Autodesk Fusion 360 part; units mm, degrees
(part 7 of 8)
  spline S189 degree 5 poles (12.6796, 61.4083) (12.6796, 61.409) (12.6791, 61.4272) (12.6782, 61.4629) (12.6766, 61.5161) (12.6742, 61.5869) (12.6707, 61.6745) (12.6667, 61.7622) (12.6623, 61.8499) (12.6573, 61.9376) (12.6519, 62.0254) (12.646, 62.1133) (12.6396, 62.2012) (12.6327, 62.2891) (12.6255, 62.3771) (12.6177, 62.4651) (12.6096, 62.5532) (12.601, 62.6413) (12.592, 62.7294) (12.5826, 62.8175) (12.5727, 62.9057) (12.5625, 62.9939) (12.5519, 63.0822) (12.5408, 63.1704) (12.5294, 63.2587) (12.5175, 63.347) (12.5053, 63.4353) (12.4927, 63.5237) (12.4798, 63.612) (12.4664, 63.7004) (12.4527, 63.7888) (12.4386, 63.8772) (12.4242, 63.9657) (12.4093, 64.0541) (12.3942, 64.1426) (12.3787, 64.231) (12.3628, 64.3195) (12.3466, 64.408) (12.33, 64.4965) (12.3131, 64.585) (12.2958, 64.6735) (12.2782, 64.762) (12.2603, 64.8506) (12.242, 64.9391) (12.2234, 65.0276) (12.2045, 65.1162) (12.1852, 65.2047) (12.1656, 65.2933) (12.1457, 65.3818) (12.1255, 65.4703) (12.1049, 65.5589) (12.0841, 65.6474) (12.0629, 65.736) (12.0457, 65.8068) (12.0327, 65.8599) (12.0239, 65.8954) (12.0195, 65.9131) knots 0.270845 0.270845 0.270845 0.270845 0.270845 0.270845 0.271429 0.285714 0.3 0.314286 0.328571 0.342857 0.357143 0.371429 0.385714 0.4 0.414286 0.428571 0.442857 0.457143 0.471429 0.485714 0.5 0.514286 0.528571 0.542857 0.557143 0.571429 0.585714 0.6 0.614286 0.628571 0.642857 0.657143 0.671429 0.685714 0.7 0.714286 0.728571 0.742857 0.757143 0.771429 0.785714 0.8 0.814286 0.828571 0.842857 0.857143 0.871429 0.885714 0.9 0.914286 0.928571 0.942857 0.957143 0.971429 0.985714 1 1 1 1 1 1
  arc A95 (12.0195, 65.9131) -> (10.5389, 66.1659) centre (0, 0) ccw
  spline S190 degree 5 poles (10.5389, 66.1659) (10.5289, 66.1507) (10.5089, 66.1202) (10.4789, 66.0744) (10.4392, 66.0133) (10.3898, 65.9368) (10.3408, 65.8602) (10.292, 65.7835) (10.2435, 65.7067) (10.1954, 65.6298) (10.1475, 65.5527) (10.0999, 65.4756) (10.0527, 65.3984) (10.0058, 65.321) (9.9592, 65.2436) (9.9129, 65.166) (9.8669, 65.0884) (9.8212, 65.0106) (9.7759, 64.9327) (9.7309, 64.8547) (9.6862, 64.7766) (9.6418, 64.6985) (9.5978, 64.6202) (9.5542, 64.5417) (9.5108, 64.4632) (9.4679, 64.3846) (9.4252, 64.3059) (9.3829, 64.227) (9.341, 64.1481) (9.2995, 64.0691) (9.2583, 63.9899) (9.2174, 63.9106) (9.177, 63.8313) (9.1369, 63.7518) (9.0971, 63.6722) (9.0578, 63.5925) (9.0189, 63.5127) (8.9803, 63.4328) (8.9422, 63.3528) (8.9045, 63.2726) (8.8671, 63.1924) (8.8302, 63.112) (8.7937, 63.0316) (8.7576, 62.951) (8.722, 62.8703) (8.6868, 62.7895) (8.6521, 62.7086) (8.6178, 62.6276) (8.584, 62.5464) (8.5507, 62.4652) (8.5178, 62.3838) (8.4854, 62.3023) (8.4597, 62.2363) (8.4406, 62.1867) (8.4278, 62.1533) (8.4213, 62.1363) (8.4211, 62.1356) knots -1 -1 -1 -1 -1 -1 -0.985714 -0.971429 -0.957143 -0.942857 -0.928571 -0.914286 -0.9 -0.885714 -0.871429 -0.857143 -0.842857 -0.828571 -0.814286 -0.8 -0.785714 -0.771429 -0.757143 -0.742857 -0.728571 -0.714286 -0.7 -0.685714 -0.671429 -0.657143 -0.642857 -0.628571 -0.614286 -0.6 -0.585714 -0.571429 -0.557143 -0.542857 -0.528571 -0.514286 -0.5 -0.485714 -0.471429 -0.457143 -0.442857 -0.428571 -0.414286 -0.4 -0.385714 -0.371429 -0.357143 -0.342857 -0.328571 -0.314286 -0.3 -0.285714 -0.271429 -0.270845 -0.270845 -0.270845 -0.270845 -0.270845 -0.270845
  spline S191 degree 3 poles (8.2079, 62.0083) (8.2337, 62.0049) (8.2599, 62.0066) (8.3103, 62.0199) (8.3339, 62.0313) (8.3696, 62.0583) (8.3829, 62.0717) (8.4054, 62.1016) (8.4144, 62.1181) (8.4211, 62.1356) knots 0 0 0 0 0.007813 0.007813 0.015626 0.015626 0.021241 0.021241 0.026855 0.026855 0.026855 0.026855
  arc A96 (8.2079, 62.0083) -> (6.8702, 62.1708) centre (0, 0) ccw
  spline S192 degree 3 poles (6.6936, 62.3453) (6.6968, 62.3195) (6.705, 62.2945) (6.7304, 62.2491) (6.7475, 62.229) (6.7825, 62.2012) (6.7988, 62.1917) (6.8334, 62.1775) (6.8516, 62.1728) (6.8702, 62.1708) knots 0 0 0 0 0.007813 0.007813 0.015626 0.015626 0.021241 0.021241 0.026855 0.026855 0.026855 0.026855
  spline S193 degree 5 poles (6.6936, 62.3453) (6.6935, 62.346) (6.6913, 62.3641) (6.687, 62.3996) (6.6803, 62.4524) (6.671, 62.5226) (6.6591, 62.6095) (6.6467, 62.6963) (6.6338, 62.7832) (6.6204, 62.8701) (6.6065, 62.957) (6.5921, 63.0438) (6.5773, 63.1307) (6.562, 63.2176) (6.5463, 63.3045) (6.5301, 63.3913) (6.5135, 63.4782) (6.4964, 63.565) (6.479, 63.6519) (6.4611, 63.7387) (6.4428, 63.8255) (6.4241, 63.9123) (6.405, 63.9991) (6.3854, 64.0859) (6.3655, 64.1726) (6.3452, 64.2594) (6.3246, 64.3461) (6.3035, 64.4328) (6.2821, 64.5195) (6.2602, 64.6062) (6.2381, 64.6929) (6.2155, 64.7795) (6.1926, 64.8661) (6.1693, 64.9527) (6.1457, 65.0393) (6.1217, 65.1259) (6.0973, 65.2124) (6.0726, 65.2989) (6.0476, 65.3854) (6.0222, 65.4719) (5.9965, 65.5583) (5.9704, 65.6447) (5.9441, 65.7311) (5.9173, 65.8175) (5.8903, 65.9038) (5.8629, 65.9901) (5.8352, 66.0764) (5.8071, 66.1626) (5.7788, 66.2488) (5.7501, 66.335) (5.7211, 66.4211) (5.6918, 66.5073) (5.6621, 66.5933) (5.6382, 66.6622) (5.6201, 66.7138) (5.608, 66.7482) (5.6019, 66.7654) knots 0.270845 0.270845 0.270845 0.270845 0.270845 0.270845 0.271429 0.285714 0.3 0.314286 0.328571 0.342857 0.357143 0.371429 0.385714 0.4 0.414286 0.428571 0.442857 0.457143 0.471429 0.485714 0.5 0.514286 0.528571 0.542857 0.557143 0.571429 0.585714 0.6 0.614286 0.628571 0.642857 0.657143 0.671429 0.685714 0.7 0.714286 0.728571 0.742857 0.757143 0.771429 0.785714 0.8 0.814286 0.828571 0.842857 0.857143 0.871429 0.885714 0.9 0.914286 0.928571 0.942857 0.957143 0.971429 0.985714 1 1 1 1 1 1
  arc A97 (5.6019, 66.7654) -> (4.1038, 66.8742) centre (0, 0) ccw
  spline S194 degree 5 poles (4.1038, 66.8742) (4.0953, 66.8581) (4.0783, 66.8258) (4.0529, 66.7773) (4.0193, 66.7127) (3.9775, 66.6318) (3.9361, 66.5508) (3.8949, 66.4697) (3.8541, 66.3886) (3.8136, 66.3074) (3.7734, 66.2261) (3.7335, 66.1447) (3.6939, 66.0633) (3.6547, 65.9818) (3.6157, 65.9002) (3.5771, 65.8185) (3.5389, 65.7368) (3.5009, 65.655) (3.4633, 65.5731) (3.4261, 65.4911) (3.3891, 65.4091) (3.3525, 65.327) (3.3163, 65.2448) (3.2804, 65.1626) (3.2448, 65.0802) (3.2097, 64.9978) (3.1748, 64.9153) (3.1403, 64.8328) (3.1062, 64.7502) (3.0725, 64.6675) (3.0391, 64.5847) (3.0061, 64.5019) (2.9735, 64.419) (2.9413, 64.336) (2.9094, 64.253) (2.878, 64.1698) (2.8469, 64.0866) (2.8163, 64.0034) (2.786, 63.9201) (2.7562, 63.8367) (2.7268, 63.7532) (2.6978, 63.6696) (2.6692, 63.586) (2.6411, 63.5024) (2.6134, 63.4186) (2.5862, 63.3348) (2.5594, 63.2509) (2.5331, 63.1669) (2.5073, 63.0829) (2.482, 62.9988) (2.4571, 62.9146) (2.4328, 62.8304) (2.4135, 62.7623) (2.3993, 62.711) (2.3898, 62.6765) (2.385, 62.659) (2.3848, 62.6583) knots -1 -1 -1 -1 -1 -1 -0.985714 -0.971429 -0.957143 -0.942857 -0.928571 -0.914286 -0.9 -0.885714 -0.871429 -0.857143 -0.842857 -0.828571 -0.814286 -0.8 -0.785714 -0.771429 -0.757143 -0.742857 -0.728571 -0.714286 -0.7 -0.685714 -0.671429 -0.657143 -0.642857 -0.628571 -0.614286 -0.6 -0.585714 -0.571429 -0.557143 -0.542857 -0.528571 -0.514286 -0.5 -0.485714 -0.471429 -0.457143 -0.442857 -0.428571 -0.414286 -0.4 -0.385714 -0.371429 -0.357143 -0.342857 -0.328571 -0.314286 -0.3 -0.285714 -0.271429 -0.270845 -0.270845 -0.270845 -0.270845 -0.270845 -0.270845
  spline S195 degree 3 poles (2.1849, 62.511) (2.2109, 62.5101) (2.2369, 62.5143) (2.2857, 62.5324) (2.3081, 62.5461) (2.3411, 62.5764) (2.353, 62.591) (2.3725, 62.6229) (2.3799, 62.6402) (2.3848, 62.6583) knots 0 0 0 0 0.007813 0.007813 0.015626 0.015626 0.021241 0.021241 0.026855 0.026855 0.026855 0.026855
  arc A98 (2.1849, 62.511) -> (0.8378, 62.5436) centre (0, 0) ccw
  spline S196 degree 3 poles (0.6452, 62.7003) (0.6508, 62.6749) (0.6614, 62.6508) (0.6911, 62.608) (0.71, 62.5898) (0.7476, 62.5655) (0.7646, 62.5576) (0.8005, 62.5467) (0.8191, 62.5438) (0.8378, 62.5436) knots 0 0 0 0 0.007813 0.007813 0.015626 0.015626 0.021241 0.021241 0.026855 0.026855 0.026855 0.026855
  spline S197 degree 5 poles (0.6452, 62.7003) (0.645, 62.701) (0.6411, 62.7188) (0.6333, 62.7537) (0.6215, 62.8056) (0.6056, 62.8746) (0.5853, 62.9599) (0.5646, 63.0452) (0.5434, 63.1304) (0.5216, 63.2156) (0.4994, 63.3007) (0.4767, 63.3858) (0.4536, 63.4708) (0.43, 63.5558) (0.4059, 63.6407) (0.3815, 63.7256) (0.3565, 63.8105) (0.3312, 63.8953) (0.3054, 63.98) (0.2792, 64.0647) (0.2526, 64.1494) (0.2257, 64.2339) (0.1983, 64.3185) (0.1705, 64.403) (0.1423, 64.4874) (0.1137, 64.5718) (0.0847, 64.6561) (0.0554, 64.7404) (0.0257, 64.8246) (-0.0044, 64.9088) (-0.0348, 64.9929) (-0.0656, 65.077) (-0.0968, 65.161) (-0.1283, 65.2449) (-0.1602, 65.3288) (-0.1925, 65.4127) (-0.225, 65.4965) (-0.258, 65.5802) (-0.2912, 65.6638) (-0.3248, 65.7475) (-0.3588, 65.831) (-0.3931, 65.9145) (-0.4277, 65.9979) (-0.4626, 66.0813) (-0.4979, 66.1646) (-0.5335, 66.2479) (-0.5694, 66.3311) (-0.6056, 66.4142) (-0.6421, 66.4973) (-0.679, 66.5803) (-0.7162, 66.6632) (-0.7537, 66.7461) (-0.7915, 66.8289) (-0.822, 66.8951) (-0.845, 66.9448) (-0.8604, 66.9778) (-0.8681, 66.9944) knots 0.270845 0.270845 0.270845 0.270845 0.270845 0.270845 0.271429 0.285714 0.3 0.314286 0.328571 0.342857 0.357143 0.371429 0.385714 0.4 0.414286 0.428571 0.442857 0.457143 0.471429 0.485714 0.5 0.514286 0.528571 0.542857 0.557143 0.571429 0.585714 0.6 0.614286 0.628571 0.642857 0.657143 0.671429 0.685714 0.7 0.714286 0.728571 0.742857 0.757143 0.771429 0.785714 0.8 0.814286 0.828571 0.842857 0.857143 0.871429 0.885714 0.9 0.914286 0.928571 0.942857 0.957143 0.971429 0.985714 1 1 1 1 1 1
  arc A99 (-0.8681, 66.9944) -> (-2.3697, 66.9581) centre (0, 0) ccw
  spline S198 degree 5 poles (-2.3697, 66.9581) (-2.3766, 66.9412) (-2.3904, 66.9074) (-2.4109, 66.8567) (-2.4382, 66.7891) (-2.4719, 66.7046) (-2.5054, 66.62) (-2.5385, 66.5353) (-2.5713, 66.4506) (-2.6038, 66.3659) (-2.636, 66.2811) (-2.6678, 66.1963) (-2.6994, 66.1114) (-2.7306, 66.0265) (-2.7614, 65.9415) (-2.792, 65.8565) (-2.8222, 65.7715) (-2.852, 65.6864) (-2.8816, 65.6012) (-2.9107, 65.5161) (-2.9396, 65.4308) (-2.9681, 65.3456) (-2.9962, 65.2603) (-3.024, 65.175) (-3.0515, 65.0896) (-3.0785, 65.0042) (-3.1052, 64.9187) (-3.1316, 64.8332) (-3.1576, 64.7477) (-3.1832, 64.6621) (-3.2084, 64.5765) (-3.2332, 64.4909) (-3.2577, 64.4052) (-3.2818, 64.3195) (-3.3055, 64.2338) (-3.3287, 64.148) (-3.3516, 64.0622) (-3.3741, 63.9764) (-3.3962, 63.8905) (-3.4178, 63.8047) (-3.439, 63.7187) (-3.4598, 63.6328) (-3.4802, 63.5468) (-3.5001, 63.4608) (-3.5196, 63.3748) (-3.5386, 63.2887) (-3.5571, 63.2026) (-3.5752, 63.1165) (-3.5928, 63.0304) (-3.6099, 62.9443) (-3.6265, 62.8581) (-3.6426, 62.7719) (-3.6552, 62.7022) (-3.6644, 62.6498) (-3.6705, 62.6146) (-3.6736, 62.5966) (-3.6737, 62.5959) knots -1 -1 -1 -1 -1 -1 -0.985714 -0.971429 -0.957143 -0.942857 -0.928571 -0.914286 -0.9 -0.885714 -0.871429 -0.857143 -0.842857 -0.828571 -0.814286 -0.8 -0.785714 -0.771429 -0.757143 -0.742857 -0.728571 -0.714286 -0.7 -0.685714 -0.671429 -0.657143 -0.642857 -0.628571 -0.614286 -0.6 -0.585714 -0.571429 -0.557143 -0.542857 -0.528571 -0.514286 -0.5 -0.485714 -0.471429 -0.457143 -0.442857 -0.428571 -0.414286 -0.4 -0.385714 -0.371429 -0.357143 -0.342857 -0.328571 -0.314286 -0.3 -0.285714 -0.271429 -0.270845 -0.270845 -0.270845 -0.270845 -0.270845 -0.270845
  spline S199 degree 3 poles (-3.8585, 62.4301) (-3.8325, 62.4317) (-3.8071, 62.4384) (-3.7602, 62.4611) (-3.7392, 62.4769) (-3.7093, 62.5102) (-3.6989, 62.5259) (-3.6826, 62.5596) (-3.6769, 62.5775) (-3.6737, 62.5959) knots 0 0 0 0 0.007813 0.007813 0.015626 0.015626 0.021241 0.021241 0.026855 0.026855 0.026855 0.026855
  arc A100 (-3.8585, 62.4301) -> (-5.2025, 62.3325) centre (0, 0) ccw
  spline S200 degree 3 poles (-5.4093, 62.4699) (-5.4012, 62.4451) (-5.3884, 62.4222) (-5.3547, 62.3825) (-5.3341, 62.3661) (-5.2943, 62.3455) (-5.2766, 62.3393) (-5.2399, 62.332) (-5.2211, 62.3309) (-5.2025, 62.3325) knots 0 0 0 0 0.007813 0.007813 0.015626 0.015626 0.021241 0.021241 0.026855 0.026855 0.026855 0.026855
  spline S201 degree 5 poles (-5.4093, 62.4699) (-5.4095, 62.4706) (-5.4151, 62.4879) (-5.4262, 62.5218) (-5.443, 62.5724) (-5.4655, 62.6395) (-5.4939, 62.7225) (-5.5228, 62.8053) (-5.5521, 62.8881) (-5.582, 62.9708) (-5.6123, 63.0534) (-5.6431, 63.1359) (-5.6743, 63.2183) (-5.706, 63.3006) (-5.7382, 63.3828) (-5.7707, 63.465) (-5.8037, 63.547) (-5.8371, 63.6289) (-5.871, 63.7108) (-5.9052, 63.7926) (-5.9398, 63.8743) (-5.9749, 63.9559) (-6.0103, 64.0374) (-6.0461, 64.1188) (-6.0823, 64.2001) (-6.1189, 64.2813) (-6.1559, 64.3625) (-6.1932, 64.4435) (-6.2309, 64.5245) (-6.269, 64.6054) (-6.3074, 64.6862) (-6.3462, 64.7668) (-6.3853, 64.8475) (-6.4248, 64.928) (-6.4646, 65.0084) (-6.5048, 65.0887) (-6.5453, 65.169) (-6.5862, 65.2491) (-6.6273, 65.3292) (-6.6689, 65.4092) (-6.7107, 65.4891) (-6.7529, 65.5688) (-6.7954, 65.6485) (-6.8382, 65.7282) (-6.8813, 65.8077) (-6.9248, 65.8871) (-6.9686, 65.9665) (-7.0127, 66.0457) (-7.0571, 66.1249) (-7.1018, 66.2039) (-7.1468, 66.2829) (-7.1921, 66.3618) (-7.2377, 66.4406) (-7.2744, 66.5035) (-7.3021, 66.5507) (-7.3206, 66.5821) (-7.3299, 66.5978) knots 0.270845 0.270845 0.270845 0.270845 0.270845 0.270845 0.271429 0.285714 0.3 0.314286 0.328571 0.342857 0.357143 0.371429 0.385714 0.4 0.414286 0.428571 0.442857 0.457143 0.471429 0.485714 0.5 0.514286 0.528571 0.542857 0.557143 0.571429 0.585714 0.6 0.614286 0.628571 0.642857 0.657143 0.671429 0.685714 0.7 0.714286 0.728571 0.742857 0.757143 0.771429 0.785714 0.8 0.814286 0.828571 0.842857 0.857143 0.871429 0.885714 0.9 0.914286 0.928571 0.942857 0.957143 0.971429 0.985714 1 1 1 1 1 1
  arc A101 (-7.3299, 66.5978) -> (-8.821, 66.4168) centre (0, 0) ccw
  spline S202 degree 5 poles (-8.821, 66.4168) (-8.8262, 66.3993) (-8.8367, 66.3644) (-8.8523, 66.3119) (-8.8729, 66.242) (-8.8983, 66.1546) (-8.9234, 66.0672) (-8.9482, 65.9797) (-8.9727, 65.8923) (-8.9969, 65.8048) (-9.0207, 65.7173) (-9.0442, 65.6298) (-9.0674, 65.5422) (-9.0903, 65.4547) (-9.1128, 65.3672) (-9.135, 65.2796) (-9.1568, 65.192) (-9.1784, 65.1045) (-9.1995, 65.0169) (-9.2204, 64.9293) (-9.2408, 64.8417) (-9.261, 64.7541) (-9.2808, 64.6665) (-9.3002, 64.5788) (-9.3193, 64.4912) (-9.338, 64.4036) (-9.3563, 64.3159) (-9.3743, 64.2283) (-9.3919, 64.1407) (-9.4091, 64.053) (-9.426, 63.9654) (-9.4424, 63.8778) (-9.4585, 63.7902) (-9.4742, 63.7025) (-9.4895, 63.6149) (-9.5044, 63.5273) (-9.5189, 63.4397) (-9.533, 63.3521) (-9.5466, 63.2645) (-9.5599, 63.1769) (-9.5727, 63.0894) (-9.5851, 63.0018) (-9.5971, 62.9143) (-9.6086, 62.8267) (-9.6197, 62.7392) (-9.6303, 62.6517) (-9.6404, 62.5643) (-9.6501, 62.4768) (-9.6593, 62.3894) (-9.668, 62.302) (-9.6762, 62.2146) (-9.6839, 62.1273) (-9.6897, 62.0567) (-9.6939, 62.0036) (-9.6965, 61.968) (-9.6979, 61.9499) (-9.6979, 61.9491) knots -1 -1 -1 -1 -1 -1 -0.985714 -0.971429 -0.957143 -0.942857 -0.928571 -0.914286 -0.9 -0.885714 -0.871429 -0.857143 -0.842857 -0.828571 -0.814286 -0.8 -0.785714 -0.771429 -0.757143 -0.742857 -0.728571 -0.714286 -0.7 -0.685714 -0.671429 -0.657143 -0.642857 -0.628571 -0.614286 -0.6 -0.585714 -0.571429 -0.557143 -0.542857 -0.528571 -0.514286 -0.5 -0.485714 -0.471429 -0.457143 -0.442857 -0.428571 -0.414286 -0.4 -0.385714 -0.371429 -0.357143 -0.342857 -0.328571 -0.314286 -0.3 -0.285714 -0.271429 -0.270845 -0.270845 -0.270845 -0.270845 -0.270845 -0.270845
  spline S203 degree 3 poles (-9.8659, 61.7662) (-9.8401, 61.7703) (-9.8155, 61.7794) (-9.771, 61.8066) (-9.7516, 61.8243) (-9.7251, 61.8604) (-9.7162, 61.877) (-9.7033, 61.9121) (-9.6993, 61.9305) (-9.6979, 61.9491) knots 0 0 0 0 0.007813 0.007813 0.015626 0.015626 0.021241 0.021241 0.026855 0.026855 0.026855 0.026855
  arc A102 (-9.8659, 61.7662) -> (-11.1941, 61.5394) centre (0, 0) ccw
  spline S204 degree 3 poles (-11.4132, 61.6562) (-11.4028, 61.6323) (-11.3878, 61.6107) (-11.3505, 61.5744) (-11.3284, 61.5601) (-11.2868, 61.5435) (-11.2686, 61.539) (-11.2313, 61.5353) (-11.2125, 61.536) (-11.1941, 61.5394) knots 0 0 0 0 0.007813 0.007813 0.015626 0.015626 0.021241 0.021241 0.026855 0.026855 0.026855 0.026855
  spline S205 degree 5 poles (-11.4132, 61.6562) (-11.4135, 61.6568) (-11.4208, 61.6735) (-11.4351, 61.7062) (-11.4567, 61.7549) (-11.4856, 61.8196) (-11.5218, 61.8994) (-11.5586, 61.9791) (-11.5958, 62.0587) (-11.6335, 62.1381) (-11.6716, 62.2174) (-11.7102, 62.2965) (-11.7493, 62.3755) (-11.7888, 62.4544) (-11.8287, 62.5331) (-11.869, 62.6117) (-11.9098, 62.6902) (-11.951, 62.7685) (-11.9925, 62.8468) (-12.0345, 62.9248) (-12.0769, 63.0028) (-12.1196, 63.0806) (-12.1627, 63.1583) (-12.2063, 63.2359) (-12.2501, 63.3134) (-12.2944, 63.3907) (-12.339, 63.4679) (-12.384, 63.545) (-12.4293, 63.6219) (-12.475, 63.6987) (-12.5211, 63.7754) (-12.5674, 63.852) (-12.6142, 63.9285) (-12.6612, 64.0048) (-12.7087, 64.081) (-12.7564, 64.1571) (-12.8045, 64.233) (-12.8529, 64.3089) (-12.9016, 64.3846) (-12.9506, 64.4602) (-13, 64.5356) (-13.0497, 64.611) (-13.0997, 64.6862) (-13.15, 64.7613) (-13.2006, 64.8363) (-13.2515, 64.9112) (-13.3027, 64.9859) (-13.3543, 65.0606) (-13.4061, 65.1351) (-13.4582, 65.2094) (-13.5106, 65.2837) (-13.5633, 65.3578) (-13.6163, 65.4319) (-13.659, 65.491) (-13.6911, 65.5353) (-13.7126, 65.5648) (-13.7233, 65.5795) knots 0.270845 0.270845 0.270845 0.270845 0.270845 0.270845 0.271429 0.285714 0.3 0.314286 0.328571 0.342857 0.357143 0.371429 0.385714 0.4 0.414286 0.428571 0.442857 0.457143 0.471429 0.485714 0.5 0.514286 0.528571 0.542857 0.557143 0.571429 0.585714 0.6 0.614286 0.628571 0.642857 0.657143 0.671429 0.685714 0.7 0.714286 0.728571 0.742857 0.757143 0.771429 0.785714 0.8 0.814286 0.828571 0.842857 0.857143 0.871429 0.885714 0.9 0.914286 0.928571 0.942857 0.957143 0.971429 0.985714 1 1 1 1 1 1
  arc A103 (-13.7233, 65.5795) -> (-15.19, 65.2554) centre (0, 0) ccw
  spline S206 degree 5 poles (-15.19, 65.2554) (-15.1935, 65.2375) (-15.2005, 65.2017) (-15.211, 65.148) (-15.2247, 65.0764) (-15.2416, 64.987) (-15.2582, 64.8975) (-15.2744, 64.8081) (-15.2903, 64.7187) (-15.306, 64.6292) (-15.3212, 64.5399) (-15.3362, 64.4505) (-15.3508, 64.3611) (-15.3651, 64.2718) (-15.3791, 64.1825) (-15.3927, 64.0932) (-15.406, 64.0039) (-15.419, 63.9147) (-15.4316, 63.8255) (-15.4439, 63.7363) (-15.4558, 63.6471) (-15.4674, 63.558) (-15.4786, 63.4688) (-15.4895, 63.3798) (-15.5, 63.2907) (-15.5102, 63.2017) (-15.52, 63.1127) (-15.5294, 63.0237) (-15.5385, 62.9348) (-15.5472, 62.8459) (-15.5555, 62.7571) (-15.5634, 62.6683) (-15.571, 62.5795) (-15.5781, 62.4908) (-15.5849, 62.4021) (-15.5913, 62.3134) (-15.5973, 62.2248) (-15.6028, 62.1363) (-15.608, 62.0478) (-15.6127, 61.9593) (-15.617, 61.8709) (-15.6209, 61.7826) (-15.6244, 61.6943) (-15.6274, 61.6061) (-15.63, 61.5179) (-15.6321, 61.4298) (-15.6338, 61.3418) (-15.6349, 61.2538) (-15.6357, 61.1659) (-15.6359, 61.0781) (-15.6356, 60.9903) (-15.6349, 60.9026) (-15.6338, 60.8318) (-15.6328, 60.7786) (-15.6321, 60.7429) (-15.6316, 60.7247) (-15.6316, 60.724) knots -1 -1 -1 -1 -1 -1 -0.985714 -0.971429 -0.957143 -0.942857 -0.928571 -0.914286 -0.9 -0.885714 -0.871429 -0.857143 -0.842857 -0.828571 -0.814286 -0.8 -0.785714 -0.771429 -0.757143 -0.742857 -0.728571 -0.714286 -0.7 -0.685714 -0.671429 -0.657143 -0.642857 -0.628571 -0.614286 -0.6 -0.585714 -0.571429 -0.557143 -0.542857 -0.528571 -0.514286 -0.5 -0.485714 -0.471429 -0.457143 -0.442857 -0.428571 -0.414286 -0.4 -0.385714 -0.371429 -0.357143 -0.342857 -0.328571 -0.314286 -0.3 -0.285714 -0.271429 -0.270845 -0.270845 -0.270845 -0.270845 -0.270845 -0.270845
  spline S207 degree 3 poles (-15.7811, 60.5257) (-15.7559, 60.5323) (-15.7322, 60.5437) (-15.6906, 60.575) (-15.673, 60.5945) (-15.6501, 60.633) (-15.6429, 60.6504) (-15.6334, 60.6866) (-15.6312, 60.7052) (-15.6316, 60.724) knots 0 0 0 0 0.007813 0.007813 0.015626 0.015626 0.021241 0.021241 0.026855 0.026855 0.026855 0.026855
  arc A104 (-15.7811, 60.5257) -> (-17.0813, 60.1717) centre (0, 0) ccw
  spline S208 degree 3 poles (-17.3106, 60.2668) (-17.298, 60.244) (-17.281, 60.224) (-17.2403, 60.1915) (-17.2169, 60.1794) (-17.174, 60.1669) (-17.1553, 60.1642) (-17.1179, 60.164) (-17.0993, 60.1666) (-17.0813, 60.1717) knots 0 0 0 0 0.007813 0.007813 0.015626 0.015626 0.021241 0.021241 0.026855 0.026855 0.026855 0.026855
  spline S209 degree 5 poles (-17.3106, 60.2668) (-17.311, 60.2674) (-17.3198, 60.2833) (-17.3373, 60.3145) (-17.3634, 60.3609) (-17.3984, 60.4225) (-17.4422, 60.4984) (-17.4865, 60.5742) (-17.5312, 60.6498) (-17.5764, 60.7252) (-17.622, 60.8004) (-17.6681, 60.8755) (-17.7145, 60.9503) (-17.7615, 61.025) (-17.8088, 61.0995) (-17.8565, 61.1739) (-17.9047, 61.2481) (-17.9532, 61.3221) (-18.0021, 61.3959) (-18.0514, 61.4696) (-18.1011, 61.5431) (-18.1512, 61.6164) (-18.2016, 61.6896) (-18.2524, 61.7626) (-18.3036, 61.8355) (-18.3551, 61.9082) (-18.4069, 61.9807) (-18.4591, 62.0531) (-18.5117, 62.1253) (-18.5646, 62.1973) (-18.6178, 62.2692) (-18.6714, 62.341) (-18.7253, 62.4126) (-18.7795, 62.484) (-18.834, 62.5553) (-18.8889, 62.6264) (-18.9441, 62.6974) (-18.9996, 62.7682) (-19.0554, 62.8388) (-19.1115, 62.9093) (-19.1679, 62.9797) (-19.2246, 63.0499) (-19.2816, 63.12) (-19.3389, 63.1899) (-19.3966, 63.2596) (-19.4545, 63.3292) (-19.5127, 63.3987) (-19.5712, 63.468) (-19.6299, 63.5371) (-19.689, 63.6061) (-19.7483, 63.675) (-19.808, 63.7437) (-19.8679, 63.8122) (-19.916, 63.867) (-19.9522, 63.9079) (-19.9765, 63.9352) (-19.9886, 63.9489) knots 0.270845 0.270845 0.270845 0.270845 0.270845 0.270845 0.271429 0.285714 0.3 0.314286 0.328571 0.342857 0.357143 0.371429 0.385714 0.4 0.414286 0.428571 0.442857 0.457143 0.471429 0.485714 0.5 0.514286 0.528571 0.542857 0.557143 0.571429 0.585714 0.6 0.614286 0.628571 0.642857 0.657143 0.671429 0.685714 0.7 0.714286 0.728571 0.742857 0.757143 0.771429 0.785714 0.8 0.814286 0.828571 0.842857 0.857143 0.871429 0.885714 0.9 0.914286 0.928571 0.942857 0.957143 0.971429 0.985714 1 1 1 1 1 1
  arc A105 (-19.9886, 63.9489) -> (-21.4171, 63.4847) centre (0, 0) ccw
  spline S210 degree 5 poles (-21.4171, 63.4847) (-21.4189, 63.4665) (-21.4224, 63.4302) (-21.4277, 63.3758) (-21.4344, 63.3032) (-21.4426, 63.2125) (-21.4505, 63.1219) (-21.458, 63.0313) (-21.4652, 62.9408) (-21.4721, 62.8503) (-21.4787, 62.7599) (-21.485, 62.6695) (-21.4909, 62.5791) (-21.4965, 62.4888) (-21.5018, 62.3986) (-21.5068, 62.3084) (-21.5114, 62.2182) (-21.5157, 62.1282) (-21.5196, 62.0381) (-21.5232, 61.9482) (-21.5265, 61.8583) (-21.5294, 61.7684) (-21.532, 61.6786) (-21.5342, 61.5889) (-21.5361, 61.4993) (-21.5376, 61.4097) (-21.5388, 61.3202) (-21.5396, 61.2307) (-21.54, 61.1413) (-21.5401, 61.052) (-21.5398, 60.9628) (-21.5391, 60.8736) (-21.5381, 60.7845) (-21.5366, 60.6955) (-21.5348, 60.6066) (-21.5326, 60.5177) (-21.53, 60.429) (-21.527, 60.3403) (-21.5236, 60.2517) (-21.5198, 60.1632) (-21.5155, 60.0748) (-21.5109, 59.9865) (-21.5058, 59.8983) (-21.5003, 59.8102) (-21.4943, 59.7222) (-21.488, 59.6343) (-21.4811, 59.5465) (-21.4738, 59.4588) (-21.466, 59.3713) (-21.4578, 59.2838) (-21.449, 59.1965) (-21.4398, 59.1093) (-21.432, 59.039) (-21.4258, 58.9861) (-21.4216, 58.9506) (-21.4194, 58.9325) (-21.4193, 58.9318) knots -1 -1 -1 -1 -1 -1 -0.985714 -0.971429 -0.957143 -0.942857 -0.928571 -0.914286 -0.9 -0.885714 -0.871429 -0.857143 -0.842857 -0.828571 -0.814286 -0.8 -0.785714 -0.771429 -0.757143 -0.742857 -0.728571 -0.714286 -0.7 -0.685714 -0.671429 -0.657143 -0.642857 -0.628571 -0.614286 -0.6 -0.585714 -0.571429 -0.557143 -0.542857 -0.528571 -0.514286 -0.5 -0.485714 -0.471429 -0.457143 -0.442857 -0.428571 -0.414286 -0.4 -0.385714 -0.371429 -0.357143 -0.342857 -0.328571 -0.314286 -0.3 -0.285714 -0.271429 -0.270845 -0.270845 -0.270845 -0.270845 -0.270845 -0.270845
  spline S211 degree 3 poles (-21.549, 58.72) (-21.5245, 58.729) (-21.5021, 58.7427) (-21.4637, 58.7778) (-21.4481, 58.799) (-21.429, 58.8395) (-21.4234, 58.8575) (-21.4175, 58.8944) (-21.4171, 58.9132) (-21.4193, 58.9318) knots 0 0 0 0 0.007813 0.007813 0.015626 0.015626 0.021241 0.021241 0.026855 0.026855 0.026855 0.026855
  arc A106 (-21.549, 58.72) -> (-22.8089, 58.2422) centre (0, 0) ccw
  spline S212 degree 3 poles (-23.0464, 58.3147) (-23.0316, 58.2933) (-23.0128, 58.275) (-22.9691, 58.2466) (-22.9447, 58.2368) (-22.9007, 58.2284) (-22.8819, 58.2276) (-22.8447, 58.231) (-22.8264, 58.2354) (-22.8089, 58.2422) knots 0 0 0 0 0.007813 0.007813 0.015626 0.015626 0.021241 0.021241 0.026855 0.026855 0.026855 0.026855
  spline S213 degree 5 poles (-23.0464, 58.3147) (-23.0468, 58.3153) (-23.0572, 58.3303) (-23.0775, 58.3597) (-23.108, 58.4033) (-23.1488, 58.4612) (-23.1997, 58.5326) (-23.2511, 58.6037) (-23.3029, 58.6747) (-23.3551, 58.7453) (-23.4078, 58.8158) (-23.4609, 58.8861) (-23.5144, 58.9561) (-23.5683, 59.0259) (-23.6226, 59.0955) (-23.6773, 59.1649) (-23.7324, 59.2341) (-23.7878, 59.3031) (-23.8437, 59.3718) (-23.8998, 59.4404) (-23.9564, 59.5088) (-24.0133, 59.5769) (-24.0706, 59.6449) (-24.1282, 59.7127) (-24.1861, 59.7803) (-24.2444, 59.8476) (-24.303, 59.9148) (-24.362, 59.9818) (-24.4212, 60.0486) (-24.4808, 60.1152) (-24.5408, 60.1817) (-24.601, 60.2479) (-24.6615, 60.314) (-24.7224, 60.3798) (-24.7836, 60.4455) (-24.845, 60.511) (-24.9068, 60.5763) (-24.9689, 60.6414) (-25.0312, 60.7064) (-25.0939, 60.7711) (-25.1568, 60.8357) (-25.2201, 60.9001) (-25.2836, 60.9643) (-25.3474, 61.0284) (-25.4114, 61.0922) (-25.4758, 61.1559) (-25.5404, 61.2194) (-25.6053, 61.2828) (-25.6705, 61.3459) (-25.736, 61.4089) (-25.8017, 61.4717) (-25.8676, 61.5343) (-25.9339, 61.5968) (-25.9871, 61.6466) (-26.0271, 61.6839) (-26.0538, 61.7087) (-26.0672, 61.7211) knots 0.270845 0.270845 0.270845 0.270845 0.270845 0.270845 0.271429 0.285714 0.3 0.314286 0.328571 0.342857 0.357143 0.371429 0.385714 0.4 0.414286 0.428571 0.442857 0.457143 0.471429 0.485714 0.5 0.514286 0.528571 0.542857 0.557143 0.571429 0.585714 0.6 0.614286 0.628571 0.642857 0.657143 0.671429 0.685714 0.7 0.714286 0.728571 0.742857 0.757143 0.771429 0.785714 0.8 0.814286 0.828571 0.842857 0.857143 0.871429 0.885714 0.9 0.914286 0.928571 0.942857 0.957143 0.971429 0.985714 1 1 1 1 1 1
  arc A107 (-26.0672, 61.7211) -> (-27.4443, 61.1213) centre (0, 0) ccw
  spline S214 degree 5 poles (-27.4443, 61.1213) (-27.4443, 61.103) (-27.4443, 61.0666) (-27.4443, 61.0119) (-27.444, 60.939) (-27.4434, 60.8479) (-27.4425, 60.757) (-27.4412, 60.6661) (-27.4397, 60.5753) (-27.4378, 60.4845) (-27.4356, 60.3939) (-27.4331, 60.3033) (-27.4303, 60.2128) (-27.4272, 60.1224) (-27.4238, 60.032) (-27.42, 59.9418) (-27.4159, 59.8516) (-27.4115, 59.7616) (-27.4067, 59.6716) (-27.4016, 59.5817) (-27.3962, 59.4919) (-27.3904, 59.4022) (-27.3843, 59.3126) (-27.3779, 59.223) (-27.3711, 59.1336) (-27.364, 59.0443) (-27.3565, 58.9551) (-27.3487, 58.866) (-27.3405, 58.777) (-27.3319, 58.6881) (-27.323, 58.5993) (-27.3137, 58.5106) (-27.3041, 58.422) (-27.2941, 58.3336) (-27.2837, 58.2452) (-27.2729, 58.157) (-27.2617, 58.0689) (-27.2502, 57.981) (-27.2382, 57.8931) (-27.2259, 57.8054) (-27.2131, 57.7178) (-27.2, 57.6304) (-27.1864, 57.5431) (-27.1724, 57.4559) (-27.158, 57.3689) (-27.1432, 57.282) (-27.1279, 57.1953) (-27.1122, 57.1087) (-27.096, 57.0223) (-27.0793, 56.9361) (-27.0622, 56.85) (-27.0446, 56.7641) (-27.03, 56.6949) (-27.0188, 56.6428) (-27.0112, 56.6079) (-27.0072, 56.5901) (-27.0071, 56.5894) knots -1 -1 -1 -1 -1 -1 -0.985714 -0.971429 -0.957143 -0.942857 -0.928571 -0.914286 -0.9 -0.885714 -0.871429 -0.857143 -0.842857 -0.828571 -0.814286 -0.8 -0.785714 -0.771429 -0.757143 -0.742857 -0.728571 -0.714286 -0.7 -0.685714 -0.671429 -0.657143 -0.642857 -0.628571 -0.614286 -0.6 -0.585714 -0.571429 -0.557143 -0.542857 -0.528571 -0.514286 -0.5 -0.485714 -0.471429 -0.457143 -0.442857 -0.428571 -0.414286 -0.4 -0.385714 -0.371429 -0.357143 -0.342857 -0.328571 -0.314286 -0.3 -0.285714 -0.271429 -0.270845 -0.270845 -0.270845 -0.270845 -0.270845 -0.270845
  spline S215 degree 3 poles (-27.1157, 56.3661) (-27.0922, 56.3774) (-27.0712, 56.3932) (-27.0363, 56.4319) (-27.0229, 56.4545) (-27.0078, 56.4966) (-27.004, 56.515) (-27.0016, 56.5524) (-27.0031, 56.5711) (-27.0071, 56.5894) knots 0 0 0 0 0.007813 0.007813 0.015626 0.015626 0.021241 0.021241 0.026855 0.026855 0.026855 0.026855
  arc A108 (-27.1157, 56.3661) -> (-28.3236, 55.7689) centre (0, 0) ccw
  spline S216 degree 3 poles (-28.567, 55.8182) (-28.5502, 55.7983) (-28.5297, 55.7819) (-28.4835, 55.7578) (-28.4582, 55.7504) (-28.4137, 55.7464) (-28.3949, 55.7473) (-28.3581, 55.7544) (-28.3403, 55.7605) (-28.3236, 55.7689) knots 0 0 0 0 0.007813 0.007813 0.015626 0.015626 0.021241 0.021241 0.026855 0.026855 0.026855 0.026855
  spline S217 degree 5 poles (-28.567, 55.8182) (-28.5675, 55.8188) (-28.5792, 55.8327) (-28.6023, 55.8599) (-28.6369, 55.9004) (-28.683, 55.9541) (-28.7406, 56.0202) (-28.7986, 56.0861) (-28.857, 56.1517) (-28.9158, 56.217) (-28.9751, 56.2821) (-29.0347, 56.3469) (-29.0947, 56.4114) (-29.1551, 56.4757) (-29.2159, 56.5397) (-29.277, 56.6035) (-29.3385, 56.6671) (-29.4004, 56.7304) (-29.4626, 56.7934) (-29.5251, 56.8563) (-29.588, 56.9188) (-29.6512, 56.9812) (-29.7147, 57.0433) (-29.7786, 57.1052) (-29.8428, 57.1669) (-29.9073, 57.2283) (-29.9722, 57.2895) (-30.0373, 57.3505) (-30.1028, 57.4113) (-30.1685, 57.4719) (-30.2346, 57.5322) (-30.3009, 57.5923) (-30.3675, 57.6522) (-30.4345, 57.7119) (-30.5017, 57.7714) (-30.5692, 57.8306) (-30.637, 57.8897) (-30.705, 57.9485) (-30.7734, 58.0071) (-30.842, 58.0655) (-30.9109, 58.1237) (-30.98, 58.1817) (-31.0494, 58.2395) (-31.1191, 58.2971) (-31.1891, 58.3545) (-31.2593, 58.4117) (-31.3297, 58.4686) (-31.4004, 58.5254) (-31.4714, 58.582) (-31.5426, 58.6384) (-31.6141, 58.6945) (-31.6858, 58.7505) (-31.7578, 58.8063) (-31.8155, 58.8507) (-31.859, 58.884) (-31.888, 58.9061) (-31.9025, 58.9172) knots 0.270845 0.270845 0.270845 0.270845 0.270845 0.270845 0.271429 0.285714 0.3 0.314286 0.328571 0.342857 0.357143 0.371429 0.385714 0.4 0.414286 0.428571 0.442857 0.457143 0.471429 0.485714 0.5 0.514286 0.528571 0.542857 0.557143 0.571429 0.585714 0.6 0.614286 0.628571 0.642857 0.657143 0.671429 0.685714 0.7 0.714286 0.728571 0.742857 0.757143 0.771429 0.785714 0.8 0.814286 0.828571 0.842857 0.857143 0.871429 0.885714 0.9 0.914286 0.928571 0.942857 0.957143 0.971429 0.985714 1 1 1 1 1 1
  arc A109 (-31.9025, 58.9172) -> (-33.2152, 58.1872) centre (0, 0) ccw
  spline S218 degree 5 poles (-33.2152, 58.1872) (-33.2135, 58.169) (-33.21, 58.1327) (-33.2046, 58.0783) (-33.1974, 58.0058) (-33.188, 57.9152) (-33.1782, 57.8248) (-33.1682, 57.7344) (-33.1579, 57.6442) (-33.1473, 57.554) (-33.1364, 57.464) (-33.1252, 57.3741) (-33.1137, 57.2843) (-33.1018, 57.1946) (-33.0897, 57.105) (-33.0772, 57.0156) (-33.0644, 56.9262) (-33.0513, 56.837) (-33.0379, 56.7479) (-33.0242, 56.6589) (-33.0101, 56.57) (-32.9957, 56.4813) (-32.981, 56.3927) (-32.9659, 56.3042) (-32.9506, 56.2159) (-32.9348, 56.1277) (-32.9188, 56.0396) (-32.9024, 55.9516) (-32.8856, 55.8638) (-32.8685, 55.7762) (-32.8511, 55.6887) (-32.8333, 55.6013) (-32.8152, 55.5141) (-32.7967, 55.427) (-32.7778, 55.3401) (-32.7585, 55.2533) (-32.7389, 55.1667) (-32.7189, 55.0803) (-32.6986, 54.994) (-32.6778, 54.9079) (-32.6567, 54.8219) (-32.6351, 54.7362) (-32.6132, 54.6506) (-32.5909, 54.5652) (-32.5681, 54.48) (-32.545, 54.3949) (-32.5214, 54.3101) (-32.4974, 54.2254) (-32.4729, 54.141) (-32.448, 54.0568) (-32.4227, 53.9728) (-32.3969, 53.889) (-32.3757, 53.8214) (-32.3595, 53.7707) (-32.3485, 53.7367) (-32.3429, 53.7194) (-32.3427, 53.7187) knots -1 -1 -1 -1 -1 -1 -0.985714 -0.971429 -0.957143 -0.942857 -0.928571 -0.914286 -0.9 -0.885714 -0.871429 -0.857143 -0.842857 -0.828571 -0.814286 -0.8 -0.785714 -0.771429 -0.757143 -0.742857 -0.728571 -0.714286 -0.7 -0.685714 -0.671429 -0.657143 -0.642857 -0.628571 -0.614286 -0.6 -0.585714 -0.571429 -0.557143 -0.542857 -0.528571 -0.514286 -0.5 -0.485714 -0.471429 -0.457143 -0.442857 -0.428571 -0.414286 -0.4 -0.385714 -0.371429 -0.357143 -0.342857 -0.328571 -0.314286 -0.3 -0.285714 -0.271429 -0.270845 -0.270845 -0.270845 -0.270845 -0.270845 -0.270845
  spline S219 degree 3 poles (-32.4292, 53.486) (-32.407, 53.4995) (-32.3875, 53.5172) (-32.3566, 53.5591) (-32.3454, 53.5828) (-32.3344, 53.6262) (-32.3324, 53.6449) (-32.3337, 53.6824) (-32.3369, 53.7009) (-32.3427, 53.7187) knots 0 0 0 0 0.007813 0.007813 0.015626 0.015626 0.021241 0.021241 0.026855 0.026855 0.026855 0.026855
  arc A110 (-32.4292, 53.486) -> (-33.5739, 52.775) centre (0, 0) ccw
  spline S220 degree 3 poles (-33.8209, 52.8005) (-33.8022, 52.7823) (-33.7802, 52.768) (-33.7319, 52.7485) (-33.7061, 52.7436) (-33.6613, 52.7438) (-33.6427, 52.7466) (-33.6068, 52.7571) (-33.5897, 52.7649) (-33.5739, 52.775) knots 0 0 0 0 0.007813 0.007813 0.015626 0.015626 0.021241 0.021241 0.026855 0.026855 0.026855 0.026855
  spline S221 degree 5 poles (-33.8209, 52.8005) (-33.8214, 52.801) (-33.8344, 52.8137) (-33.86, 52.8386) (-33.8983, 52.8756) (-33.9495, 52.9246) (-34.0132, 52.9848) (-34.0773, 53.0448) (-34.1417, 53.1044) (-34.2066, 53.1638) (-34.2718, 53.2228) (-34.3374, 53.2816) (-34.4034, 53.34) (-34.4697, 53.3982) (-34.5364, 53.456) (-34.6034, 53.5136) (-34.6707, 53.5709) (-34.7384, 53.628) (-34.8064, 53.6847) (-34.8747, 53.7412) (-34.9433, 53.7975) (-35.0123, 53.8534) (-35.0815, 53.9091) (-35.1511, 53.9646) (-35.2209, 54.0198) (-35.2911, 54.0747) (-35.3615, 54.1294) (-35.4322, 54.1838) (-35.5032, 54.238) (-35.5745, 54.2919) (-35.6461, 54.3456) (-35.7179, 54.399) (-35.79, 54.4522) (-35.8624, 54.5051) (-35.935, 54.5578) (-36.0079, 54.6103) (-36.0811, 54.6625) (-36.1545, 54.7145) (-36.2282, 54.7662) (-36.3021, 54.8178) (-36.3763, 54.8691) (-36.4507, 54.9201) (-36.5254, 54.9709) (-36.6003, 55.0215) (-36.6755, 55.0719) (-36.7509, 55.122) (-36.8265, 55.1719) (-36.9024, 55.2216) (-36.9785, 55.2711) (-37.0548, 55.3203) (-37.1313, 55.3693) (-37.2081, 55.4181) (-37.2851, 55.4667) (-37.3469, 55.5053) (-37.3934, 55.5343) (-37.4244, 55.5535) (-37.4399, 55.5631) knots 0.270845 0.270845 0.270845 0.270845 0.270845 0.270845 0.271429 0.285714 0.3 0.314286 0.328571 0.342857 0.357143 0.371429 0.385714 0.4 0.414286 0.428571 0.442857 0.457143 0.471429 0.485714 0.5 0.514286 0.528571 0.542857 0.557143 0.571429 0.585714 0.6 0.614286 0.628571 0.642857 0.657143 0.671429 0.685714 0.7 0.714286 0.728571 0.742857 0.757143 0.771429 0.785714 0.8 0.814286 0.828571 0.842857 0.857143 0.871429 0.885714 0.9 0.914286 0.928571 0.942857 0.957143 0.971429 0.985714 1 1 1 1 1 1
  arc A111 (-37.4399, 55.5631) -> (-38.676, 54.7098) centre (0, 0) ccw
  spline S222 degree 5 poles (-38.676, 54.7098) (-38.6725, 54.6919) (-38.6656, 54.6561) (-38.655, 54.6024) (-38.6407, 54.531) (-38.6226, 54.4417) (-38.6043, 54.3526) (-38.5856, 54.2637) (-38.5666, 54.1749) (-38.5473, 54.0862) (-38.5278, 53.9976) (-38.5079, 53.9092) (-38.4878, 53.8209) (-38.4674, 53.7328) (-38.4466, 53.6448) (-38.4256, 53.557) (-38.4042, 53.4693) (-38.3826, 53.3817) (-38.3606, 53.2943) (-38.3384, 53.2071) (-38.3158, 53.12) (-38.2929, 53.0331) (-38.2697, 52.9463) (-38.2462, 52.8597) (-38.2223, 52.7733) (-38.1982, 52.687) (-38.1737, 52.6009) (-38.1489, 52.5149) (-38.1238, 52.4291) (-38.0983, 52.3435) (-38.0725, 52.2581) (-38.0463, 52.1729) (-38.0198, 52.0878) (-37.993, 52.0029) (-37.9658, 51.9182) (-37.9383, 51.8337) (-37.9104, 51.7494) (-37.8822, 51.6653) (-37.8536, 51.5814) (-37.8246, 51.4977) (-37.7953, 51.4142) (-37.7656, 51.3309) (-37.7355, 51.2478) (-37.705, 51.165) (-37.6742, 51.0823) (-37.6429, 50.9999) (-37.6113, 50.9178) (-37.5792, 50.8358) (-37.5467, 50.7542) (-37.5138, 50.6727) (-37.4804, 50.5916) (-37.4467, 50.5106) (-37.419, 50.4455) (-37.398, 50.3965) (-37.3838, 50.3637) (-37.3766, 50.347) (-37.3763, 50.3464) knots -1 -1 -1 -1 -1 -1 -0.985714 -0.971429 -0.957143 -0.942857 -0.928571 -0.914286 -0.9 -0.885714 -0.871429 -0.857143 -0.842857 -0.828571 -0.814286 -0.8 -0.785714 -0.771429 -0.757143 -0.742857 -0.728571 -0.714286 -0.7 -0.685714 -0.671429 -0.657143 -0.642857 -0.628571 -0.614286 -0.6 -0.585714 -0.571429 -0.557143 -0.542857 -0.528571 -0.514286 -0.5 -0.485714 -0.471429 -0.457143 -0.442857 -0.428571 -0.414286 -0.4 -0.385714 -0.371429 -0.357143 -0.342857 -0.328571 -0.314286 -0.3 -0.285714 -0.271429 -0.270845 -0.270845 -0.270845 -0.270845 -0.270845 -0.270845
  spline S223 degree 3 poles (-37.44, 50.1064) (-37.4191, 50.122) (-37.4015, 50.1415) (-37.3747, 50.1862) (-37.3658, 50.2109) (-37.3591, 50.2552) (-37.359, 50.274) (-37.3638, 50.3111) (-37.3688, 50.3292) (-37.3763, 50.3464) knots 0 0 0 0 0.007813 0.007813 0.015626 0.015626 0.021241 0.021241 0.026855 0.026855 0.026855 0.026855
  arc A112 (-37.44, 50.1064) -> (-38.5107, 49.2882) centre (0, 0) ccw
  spline S224 degree 3 poles (-38.759, 49.2898) (-38.7387, 49.2735) (-38.7154, 49.2614) (-38.6654, 49.2466) (-38.6392, 49.2442) (-38.5947, 49.2488) (-38.5764, 49.2533) (-38.5417, 49.2673) (-38.5254, 49.2767) (-38.5107, 49.2882) knots 0 0 0 0 0.007813 0.007813 0.015626 0.015626 0.021241 0.021241 0.026855 0.026855 0.026855 0.026855
  spline S225 degree 5 poles (-38.759, 49.2898) (-38.7595, 49.2903) (-38.7737, 49.3017) (-38.8016, 49.324) (-38.8433, 49.3571) (-38.899, 49.4009) (-38.9682, 49.4547) (-39.0377, 49.5082) (-39.1077, 49.5614) (-39.1779, 49.6142) (-39.2486, 49.6667) (-39.3195, 49.7188) (-39.3908, 49.7706) (-39.4624, 49.8221) (-39.5344, 49.8732) (-39.6066, 49.9241) (-39.6792, 49.9746) (-39.7521, 50.0249) (-39.8252, 50.0748) (-39.8987, 50.1245) (-39.9724, 50.1738) (-40.0464, 50.2229) (-40.1207, 50.2716) (-40.1953, 50.3201) (-40.2701, 50.3683) (-40.3453, 50.4162) (-40.4206, 50.4638) (-40.4963, 50.5111) (-40.5722, 50.5582) (-40.6484, 50.605) (-40.7248, 50.6515) (-40.8014, 50.6978) (-40.8783, 50.7437) (-40.9555, 50.7894) (-41.0329, 50.8349) (-41.1105, 50.8801) (-41.1884, 50.925) (-41.2665, 50.9697) (-41.3448, 51.0141) (-41.4233, 51.0582) (-41.5021, 51.1021) (-41.5811, 51.1457) (-41.6604, 51.1891) (-41.7398, 51.2322) (-41.8195, 51.2751) (-41.8994, 51.3177) (-41.9795, 51.3601) (-42.0598, 51.4022) (-42.1403, 51.4441) (-42.221, 51.4857) (-42.3019, 51.5271) (-42.383, 51.5683) (-42.4644, 51.6092) (-42.5296, 51.6417) (-42.5786, 51.666) (-42.6113, 51.6822) (-42.6277, 51.6902) knots 0.270845 0.270845 0.270845 0.270845 0.270845 0.270845 0.271429 0.285714 0.3 0.314286 0.328571 0.342857 0.357143 0.371429 0.385714 0.4 0.414286 0.428571 0.442857 0.457143 0.471429 0.485714 0.5 0.514286 0.528571 0.542857 0.557143 0.571429 0.585714 0.6 0.614286 0.628571 0.642857 0.657143 0.671429 0.685714 0.7 0.714286 0.728571 0.742857 0.757143 0.771429 0.785714 0.8 0.814286 0.828571 0.842857 0.857143 0.871429 0.885714 0.9 0.914286 0.928571 0.942857 0.957143 0.971429 0.985714 1 1 1 1 1 1
  arc A113 (-42.6277, 51.6902) -> (-43.7757, 50.7216) centre (0, 0) ccw
  spline S226 degree 5 poles (-43.7757, 50.7216) (-43.7705, 50.7042) (-43.7601, 50.6692) (-43.7444, 50.6168) (-43.7234, 50.547) (-43.6967, 50.46) (-43.6698, 50.3731) (-43.6426, 50.2863) (-43.6152, 50.1997) (-43.5875, 50.1133) (-43.5595, 50.0271) (-43.5312, 49.941) (-43.5026, 49.8551) (-43.4737, 49.7693) (-43.4446, 49.6838) (-43.4152, 49.5984) (-43.3855, 49.5131) (-43.3555, 49.4281) (-43.3252, 49.3432) (-43.2946, 49.2585) (-43.2637, 49.174) (-43.2326, 49.0897) (-43.2011, 49.0056) (-43.1693, 48.9216) (-43.1373, 48.8379) (-43.1049, 48.7544) (-43.0722, 48.671) (-43.0392, 48.5878) (-43.0059, 48.5049) (-42.9723, 48.4222) (-42.9384, 48.3396) (-42.9041, 48.2573) (-42.8696, 48.1752) (-42.8347, 48.0933) (-42.7994, 48.0116) (-42.7639, 47.9302) (-42.728, 47.8489) (-42.6918, 47.768) (-42.6552, 47.6872) (-42.6183, 47.6067) (-42.581, 47.5264) (-42.5434, 47.4464) (-42.5055, 47.3666) (-42.4671, 47.2871) (-42.4285, 47.2078) (-42.3894, 47.1288) (-42.3499, 47.0501) (-42.3101, 46.9716) (-42.2699, 46.8935) (-42.2293, 46.8156) (-42.1883, 46.738) (-42.1468, 46.6607) (-42.113, 46.5985) (-42.0874, 46.5518) (-42.0701, 46.5206) (-42.0613, 46.5046) (-42.0609, 46.504) knots -1 -1 -1 -1 -1 -1 -0.985714 -0.971429 -0.957143 -0.942857 -0.928571 -0.914286 -0.9 -0.885714 -0.871429 -0.857143 -0.842857 -0.828571 -0.814286 -0.8 -0.785714 -0.771429 -0.757143 -0.742857 -0.728571 -0.714286 -0.7 -0.685714 -0.671429 -0.657143 -0.642857 -0.628571 -0.614286 -0.6 -0.585714 -0.571429 -0.557143 -0.542857 -0.528571 -0.514286 -0.5 -0.485714 -0.471429 -0.457143 -0.442857 -0.428571 -0.414286 -0.4 -0.385714 -0.371429 -0.357143 -0.342857 -0.328571 -0.314286 -0.3 -0.285714 -0.271429 -0.270845 -0.270845 -0.270845 -0.270845 -0.270845 -0.270845
  spline S227 degree 3 poles (-42.1012, 46.259) (-42.0819, 46.2765) (-42.0662, 46.2977) (-42.0439, 46.3447) (-42.0375, 46.3702) (-42.0351, 46.4149) (-42.0367, 46.4336) (-42.0451, 46.4701) (-42.0518, 46.4877) (-42.0609, 46.504) knots 0 0 0 0 0.007813 0.007813 0.015626 0.015626 0.021241 0.021241 0.026855 0.026855 0.026855 0.026855
  arc A114 (-42.1012, 46.259) -> (-43.0879, 45.3413) centre (0, 0) ccw
  spline S228 degree 3 poles (-43.3352, 45.319) (-43.3134, 45.3047) (-43.289, 45.2948) (-43.2379, 45.285) (-43.2116, 45.2851) (-43.1677, 45.294) (-43.15, 45.3002) (-43.1168, 45.3175) (-43.1015, 45.3284) (-43.0879, 45.3413) knots 0 0 0 0 0.007813 0.007813 0.015626 0.015626 0.021241 0.021241 0.026855 0.026855 0.026855 0.026855
  spline S229 degree 5 poles (-43.3352, 45.319) (-43.3358, 45.3193) (-43.351, 45.3293) (-43.3809, 45.3488) (-43.4256, 45.3778) (-43.4852, 45.416) (-43.5593, 45.4629) (-43.6337, 45.5094) (-43.7085, 45.5556) (-43.7835, 45.6014) (-43.8589, 45.6468) (-43.9345, 45.6918) (-44.0105, 45.7365) (-44.0867, 45.7808) (-44.1633, 45.8248) (-44.2401, 45.8684) (-44.3172, 45.9118) (-44.3946, 45.9547) (-44.4722, 45.9974) (-44.5501, 46.0397) (-44.6283, 46.0817) (-44.7067, 46.1234) (-44.7853, 46.1647) (-44.8642, 46.2058) (-44.9434, 46.2465) (-45.0228, 46.2869) (-45.1024, 46.3271) (-45.1823, 46.3669) (-45.2624, 46.4064) (-45.3427, 46.4456) (-45.4232, 46.4845) (-45.504, 46.5232) (-45.585, 46.5615) (-45.6662, 46.5996) (-45.7476, 46.6373) (-45.8292, 46.6748) (-45.9111, 46.712) (-45.9931, 46.7489) (-46.0753, 46.7856) (-46.1578, 46.8219) (-46.2404, 46.858) (-46.3233, 46.8938) (-46.4063, 46.9293) (-46.4896, 46.9646) (-46.573, 46.9996) (-46.6566, 47.0343) (-46.7404, 47.0687) (-46.8244, 47.1029) (-46.9086, 47.1368) (-46.993, 47.1705) (-47.0775, 47.2039) (-47.1622, 47.237) (-47.2471, 47.2699) (-47.3152, 47.2959) (-47.3663, 47.3154) (-47.4005, 47.3283) (-47.4175, 47.3347) knots 0.270845 0.270845 0.270845 0.270845 0.270845 0.270845 0.271429 0.285714 0.3 0.314286 0.328571 0.342857 0.357143 0.371429 0.385714 0.4 0.414286 0.428571 0.442857 0.457143 0.471429 0.485714 0.5 0.514286 0.528571 0.542857 0.557143 0.571429 0.585714 0.6 0.614286 0.628571 0.642857 0.657143 0.671429 0.685714 0.7 0.714286 0.728571 0.742857 0.757143 0.771429 0.785714 0.8 0.814286 0.828571 0.842857 0.857143 0.871429 0.885714 0.9 0.914286 0.928571 0.942857 0.957143 0.971429 0.985714 1 1 1 1 1 1
  arc A115 (-47.4175, 47.3347) -> (-48.4667, 46.2599) centre (0, 0) ccw
  spline S230 degree 5 poles (-48.4667, 46.2599) (-48.4599, 46.243) (-48.4461, 46.2092) (-48.4254, 46.1585) (-48.3977, 46.0911) (-48.3628, 46.0071) (-48.3277, 45.9232) (-48.2922, 45.8394) (-48.2566, 45.7559) (-48.2206, 45.6726) (-48.1844, 45.5894) (-48.1479, 45.5065) (-48.1112, 45.4237) (-48.0742, 45.3412) (-48.037, 45.2588) (-47.9994, 45.1766) (-47.9616, 45.0947) (-47.9236, 45.0129) (-47.8852, 44.9314) (-47.8466, 44.85) (-47.8077, 44.7689) (-47.7686, 44.688) (-47.7291, 44.6073) (-47.6894, 44.5268) (-47.6494, 44.4466) (-47.6091, 44.3665) (-47.5686, 44.2867) (-47.5277, 44.2071) (-47.4866, 44.1278) (-47.4451, 44.0487) (-47.4034, 43.9698) (-47.3613, 43.8912) (-47.319, 43.8128) (-47.2764, 43.7346) (-47.2334, 43.6567) (-47.1902, 43.5791) (-47.1466, 43.5017) (-47.1027, 43.4246) (-47.0586, 43.3478) (-47.014, 43.2712) (-46.9692, 43.1949) (-46.9241, 43.1188) (-46.8786, 43.0431) (-46.8327, 42.9676) (-46.7866, 42.8925) (-46.7401, 42.8176) (-46.6932, 42.7431) (-46.646, 42.6688) (-46.5984, 42.5949) (-46.5505, 42.5213) (-46.5022, 42.4481) (-46.4535, 42.3751) (-46.4138, 42.3165) (-46.3838, 42.2725) (-46.3636, 42.243) (-46.3533, 42.228) (-46.3529, 42.2275) knots -1 -1 -1 -1 -1 -1 -0.985714 -0.971429 -0.957143 -0.942857 -0.928571 -0.914286 -0.9 -0.885714 -0.871429 -0.857143 -0.842857 -0.828571 -0.814286 -0.8 -0.785714 -0.771429 -0.757143 -0.742857 -0.728571 -0.714286 -0.7 -0.685714 -0.671429 -0.657143 -0.642857 -0.628571 -0.614286 -0.6 -0.585714 -0.571429 -0.557143 -0.542857 -0.528571 -0.514286 -0.5 -0.485714 -0.471429 -0.457143 -0.442857 -0.428571 -0.414286 -0.4 -0.385714 -0.371429 -0.357143 -0.342857 -0.328571 -0.314286 -0.3 -0.285714 -0.271429 -0.270845 -0.270845 -0.270845 -0.270845 -0.270845 -0.270845
  spline S231 degree 3 poles (-46.3693, 41.9797) (-46.3518, 41.999) (-46.3382, 42.0215) (-46.3206, 42.0705) (-46.3166, 42.0965) (-46.3185, 42.1412) (-46.3219, 42.1597) (-46.3338, 42.1952) (-46.3422, 42.212) (-46.3529, 42.2275) knots 0 0 0 0 0.007813 0.007813 0.015626 0.015626 0.021241 0.021241 0.026855 0.026855 0.026855 0.026855
  arc A116 (-46.3693, 41.9797) -> (-47.2628, 40.9711) centre (0, 0) ccw
  spline S232 degree 3 poles (-47.5068, 40.9249) (-47.4837, 40.9128) (-47.4585, 40.9054) (-47.4067, 40.9005) (-47.3805, 40.9032) (-47.3377, 40.9162) (-47.3206, 40.9242) (-47.2893, 40.9446) (-47.2751, 40.9569) (-47.2628, 40.9711) knots 0 0 0 0 0.007813 0.007813 0.015626 0.015626 0.021241 0.021241 0.026855 0.026855 0.026855 0.026855
  spline S233 degree 5 poles (-47.5068, 40.9249) (-47.5074, 40.9253) (-47.5236, 40.9337) (-47.5552, 40.9503) (-47.6025, 40.9748) (-47.6655, 41.007) (-47.7438, 41.0466) (-47.8223, 41.0857) (-47.9012, 41.1244) (-47.9803, 41.1628) (-48.0597, 41.2007) (-48.1393, 41.2382) (-48.2192, 41.2753) (-48.2994, 41.3121) (-48.3798, 41.3485) (-48.4605, 41.3845) (-48.5414, 41.4202) (-48.6226, 41.4555) (-48.704, 41.4905) (-48.7856, 41.5251) (-48.8674, 41.5593) (-48.9495, 41.5932) (-49.0318, 41.6268) (-49.1143, 41.66) (-49.197, 41.6929) (-49.2799, 41.7255) (-49.3631, 41.7578) (-49.4464, 41.7897) (-49.5299, 41.8213) (-49.6136, 41.8526) (-49.6976, 41.8836) (-49.7817, 41.9142) (-49.866, 41.9446) (-49.9505, 41.9746) (-50.0352, 42.0043) (-50.12, 42.0338) (-50.2051, 42.0629) (-50.2903, 42.0917) (-50.3757, 42.1202) (-50.4613, 42.1485) (-50.547, 42.1764) (-50.6329, 42.204) (-50.719, 42.2314) (-50.8053, 42.2584) (-50.8917, 42.2852) (-50.9783, 42.3117) (-51.065, 42.3379) (-51.1519, 42.3638) (-51.239, 42.3894) (-51.3262, 42.4148) (-51.4136, 42.4399) (-51.5011, 42.4647) (-51.5888, 42.4892) (-51.659, 42.5086) (-51.7118, 42.523) (-51.747, 42.5326) (-51.7646, 42.5373) knots 0.270845 0.270845 0.270845 0.270845 0.270845 0.270845 0.271429 0.285714 0.3 0.314286 0.328571 0.342857 0.357143 0.371429 0.385714 0.4 0.414286 0.428571 0.442857 0.457143 0.471429 0.485714 0.5 0.514286 0.528571 0.542857 0.557143 0.571429 0.585714 0.6 0.614286 0.628571 0.642857 0.657143 0.671429 0.685714 0.7 0.714286 0.728571 0.742857 0.757143 0.771429 0.785714 0.8 0.814286 0.828571 0.842857 0.857143 0.871429 0.885714 0.9 0.914286 0.928571 0.942857 0.957143 0.971429 0.985714 1 1 1 1 1 1
  arc A117 (-51.7646, 42.5373) -> (-52.7052, 41.3662) centre (0, 0) ccw
  spline S234 degree 5 poles (-52.7052, 41.3662) (-52.6967, 41.3501) (-52.6798, 41.3177) (-52.6543, 41.2693) (-52.6202, 41.2049) (-52.5774, 41.1246) (-52.5343, 41.0445) (-52.4909, 40.9646) (-52.4474, 40.8849) (-52.4035, 40.8054) (-52.3595, 40.7261) (-52.3152, 40.6471) (-52.2706, 40.5683) (-52.2259, 40.4897) (-52.1808, 40.4113) (-52.1355, 40.3331) (-52.09, 40.2552) (-52.0442, 40.1775) (-51.9982, 40.1) (-51.9519, 40.0228) (-51.9054, 39.9458) (-51.8586, 39.869) (-51.8116, 39.7925) (-51.7643, 39.7163) (-51.7167, 39.6402) (-51.6689, 39.5645) (-51.6208, 39.4889) (-51.5724, 39.4137) (-51.5238, 39.3387) (-51.4749, 39.2639) (-51.4258, 39.1894) (-51.3763, 39.1152) (-51.3266, 39.0413) (-51.2767, 38.9676) (-51.2264, 38.8942) (-51.1759, 38.8211) (-51.125, 38.7483) (-51.0739, 38.6758) (-51.0225, 38.6036) (-50.9708, 38.5317) (-50.9189, 38.46) (-50.8666, 38.3887) (-50.814, 38.3177) (-50.7611, 38.247) (-50.7079, 38.1767) (-50.6544, 38.1067) (-50.6005, 38.037) (-50.5464, 37.9676) (-50.4919, 37.8987) (-50.4371, 37.83) (-50.3819, 37.7618) (-50.3264, 37.6939) (-50.2813, 37.6393) (-50.2472, 37.5985) (-50.2242, 37.5711) (-50.2125, 37.5572) (-50.212, 37.5566) knots -1 -1 -1 -1 -1 -1 -0.985714 -0.971429 -0.957143 -0.942857 -0.928571 -0.914286 -0.9 -0.885714 -0.871429 -0.857143 -0.842857 -0.828571 -0.814286 -0.8 -0.785714 -0.771429 -0.757143 -0.742857 -0.728571 -0.714286 -0.7 -0.685714 -0.671429 -0.657143 -0.642857 -0.628571 -0.614286 -0.6 -0.585714 -0.571429 -0.557143 -0.542857 -0.528571 -0.514286 -0.5 -0.485714 -0.471429 -0.457143 -0.442857 -0.428571 -0.414286 -0.4 -0.385714 -0.371429 -0.357143 -0.342857 -0.328571 -0.314286 -0.3 -0.285714 -0.271429 -0.270845 -0.270845 -0.270845 -0.270845 -0.270845 -0.270845
  spline S235 degree 3 poles (-50.2044, 37.3084) (-50.1889, 37.3293) (-50.1776, 37.3531) (-50.1647, 37.4036) (-50.1633, 37.4298) (-50.1695, 37.4741) (-50.1747, 37.4922) (-50.19, 37.5264) (-50.1999, 37.5423) (-50.212, 37.5566) knots 0 0 0 0 0.007813 0.007813 0.015626 0.015626 0.021241 0.021241 0.026855 0.026855 0.026855 0.026855
  arc A118 (-50.2044, 37.3084) -> (-50.9965, 36.2183) centre (0, 0) ccw
  spline S236 degree 3 poles (-51.2348, 36.1488) (-51.2107, 36.139) (-51.1849, 36.134) (-51.1328, 36.1342) (-51.107, 36.1394) (-51.0657, 36.1565) (-51.0495, 36.166) (-51.0202, 36.1894) (-51.0073, 36.203) (-50.9965, 36.2183) knots 0 0 0 0 0.007813 0.007813 0.015626 0.015626 0.021241 0.021241 0.026855 0.026855 0.026855 0.026855